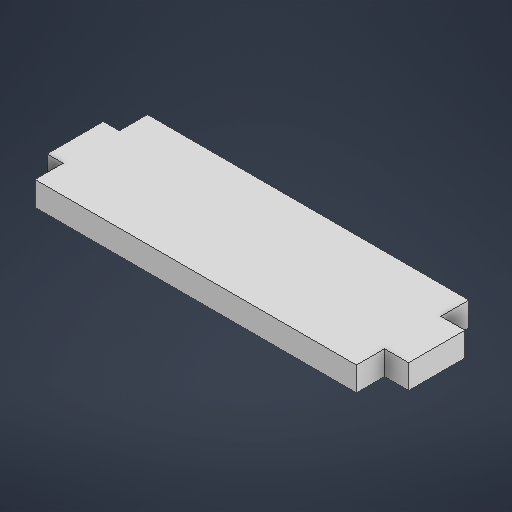
# Autodesk Inventor part: Spojka
Saved by Autodesk Inventor 2026 (Build 300175000, 175)
## iProperties
Created: 2025-06-20
Part Number: Spojka
Material: Všeobecné
Document SubType Name: Modeling
Designer: vadim
Density: 1 g/cm^3
Appearance: Výchozí
Author: vadim
Autodesk Inventor part; units mm, degrees
ref_plane "YZ Plane" through (0, 0, 0) normal (1, 0, 0) x (0, 1, 0)
ref_plane "XZ Plane" through (0, 0, 0) normal (0, 1, 0) x (-1, 0, 0)
ref_plane "XY Plane" through (0, 0, 0) normal (0, 0, 1) x (1, 0, 0)
sketch "Náčrt1" plane through (0, 0, 0) normal (0, 1, 0) x (-1, 0, 0)
  line L0 (20, 7) -> (-20, 7)
  line L1 (-20, -7) -> (20, -7)
  line L2 (20, 7) -> (-20, -7) construction
  line L3 (-20, 7) -> (20, -7) construction
  line L4 (22, -3.5) -> (20, -3.5)
  line L5 (20, 0) -> (20, 3.5)
  line L6 (20, 3.5) -> (22, 3.5)
  line L7 (22, 3.5) -> (22, -3.5)
  line L8 (22, -3.5) -> (20, 3.5) construction
  line L9 (20, -3.5) -> (22, 3.5) construction
  line L10 (20, 0) -> (-20, 0)
  line L11 (-20, 3.5) -> (-23, 3.5)
  line L12 (-23, 3.5) -> (-23, -3.5)
  line L13 (-23, -3.5) -> (-20, -3.5)
  line L14 (-20, 3.5) -> (-23, -3.5) construction
  line L15 (-23, 3.5) -> (-20, -3.5) construction
  line L16 (-20, 7) -> (-20, 3.5)
  line L17 (-20, -3.5) -> (-20, -7)
  line L18 (20, -7) -> (20, -3.5)
  line L19 (20, 0) -> (20, 7)
  point P0 (0, 0)
  point P1 (21, 0)
  point P2 (-21.5, 0)
  dimension "d0" = 14
  dimension "d2" = 7
  dimension "d5" = 7
  dimension "d7" = 45
  dimension "d8" = 2
  dimension "d9" = 3
  constraints: 40 end point, 8 parallel, 6 midpoint, 4 perpendicular, 3 horizontal, 2 collinear, 1 point on line, 1 other
  measures "d0" distance of L1.start L0.end
  measures "d2" distance of L5.end L4.end
  measures "d5" distance of L12.end L11.end
  measures "d7" distance between parallel lines of L12 L7
  measures "d8" distance between parallel lines of L19 L7
  measures "d9" distance between parallel lines of L17 L12
extrude "Vysunutí1" add sketch "Náčrt1" along normal blind 3
